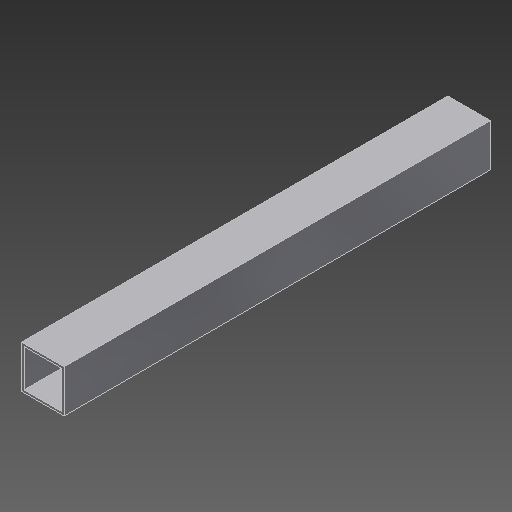
# Autodesk Inventor part: STAQ20-200
Saved by Autodesk Inventor 2021.1 (Build 251245010, 245A)
## iProperties
Created: 2010-03-11
Part Number: STAQ20-200
Material: MISUMI
Document SubType Name: Modeling
Density: 1 g/cm^3
Mass: 18.048 g
Surface Area: 302.605 cm^2
Volume: 18.048 cm^3
Appearance: Metal-Steel (Stainless, Brushed)
Title: スタンド用支柱
Autodesk Inventor part; units mm, degrees
ref_plane "YZ Plane" through (0, 0, 0) normal (1, 0, 0) x (0, 1, 0)
ref_plane "XZ Plane" through (0, 0, 0) normal (0, 1, 0) x (-1, 0, 0)
ref_plane "XY Plane" through (0, 0, 0) normal (0, 0, 1) x (1, 0, 0)
sketch "スケッチ1" plane through (0, 0, 0) normal (0, 0, 1) x (1, 0, 0)
  line L0 (-10, 10) -> (10, 10)
  line L1 (10, 10) -> (10, -10)
  line L2 (10, -10) -> (-10, -10)
  line L3 (-10, -10) -> (-10, 10)
  line L4 (8.8, 8.8) -> (-8.8, 8.8)
  line L5 (-8.8, 8.8) -> (-8.8, -8.8)
  line L6 (-8.8, -8.8) -> (8.8, -8.8)
  line L7 (8.8, -8.8) -> (8.8, 8.8)
  point P0 (0, 0)
  point P1 (-10, 0)
  point P2 (0, -10)
  dimension "d0" = 20
  dimension "d1" = 20
  dimension "d2" = 17.6
  constraints: 16 end point, 4 parallel, 2 midpoint, 2 perpendicular, 1 horizontal, 1 horizontal alignment, 1 vertical alignment, 3 other
  measures "d0" distance of L1.end L2.end
  measures "d1" distance of L2.end L0.start
  measures "d2" distance of L4.start L4.end
extrude "押し出し1" add sketch "スケッチ1" along normal blind 200
equation "\"d1\" = d0"
